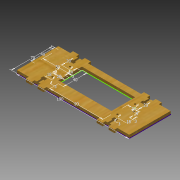
# Autodesk Inventor part: lateral_mdf2
Saved by Autodesk Inventor 2014 (Build 180170000, 170)
## iProperties
Created: 2014-11-10
Part Number: lateral_mdf2
Material: Generic
Document SubType Name: Modeling
Designer: Gabriel
Density: 1 g/cm^3
Appearance: Default
Author: Gabriel
Autodesk Inventor part; units mm, degrees
ref_plane "YZ Plane" through (0, 0, 0) normal (1, 0, 0) x (0, 1, 0)
ref_plane "XZ Plane" through (0, 0, 0) normal (0, 1, 0) x (-1, 0, 0)
ref_plane "XY Plane" through (0, 0, 0) normal (0, 0, 1) x (1, 0, 0)
sketch "Sketch1" plane through (0, 0, 0) normal (0, 0, 1) x (1, 0, 0)
  line L0 (0, 0) -> (190, 0)
  line L1 (190, 0) -> (190, -70)
  line L2 (190, -70) -> (0, -70)
  line L3 (0, -70) -> (0, 0)
  line L4 (0, 0) -> (0, -40)
  line L5 (0, 0) -> (0, -10)
  line L6 (50, -10) -> (50, -50)
  line L7 (50, -50) -> (140, -50)
  line L8 (140, -50) -> (140, -10)
  line L9 (140, -10) -> (50, -10)
  circle A0 centre (40, -20) radius 1.5
  circle A1 centre (150, -20) radius 1.5
  circle A2 centre (150, -50) radius 1.5
  circle A3 centre (40, -50) radius 1.5
  line L10 (50, -10) -> (50, -12)
  line L11 (50, -12) -> (50, -32)
  line L12 (50, -32) -> (30, -32)
  line L13 (140, -32) -> (160, -32)
  circle A4 centre (30, -32) radius 1.5
  circle A5 centre (160, -32) radius 1.5
  dimension "d0" = 190
  dimension "d1" = 70
  dimension "d116" = 40
  dimension "d118" = 50
  dimension "d119" = 40
  dimension "d120" = 90
  dimension "d125" = 3
  dimension "d126" = 3
  dimension "d127" = 3
  dimension "d128" = 3
  dimension "d130" = 20
  dimension "d131" = 20
  dimension "d132" = 20
  dimension "d133" = 3
  dimension "d134" = 3
  dimension "d140" = 20
  dimension "d141" = 20
  dimension "d145" = 18
  dimension "d146" = 18
  constraints: 28 end point, 6 centre point, 5 point on line, 4 parallel, 2 coincident, 2 perpendicular, 1 collinear, 1 horizontal
  measures "d0" distance of L1.end L2.end
  measures "d1" distance of L2.end L0.start
  measures "d116" distance of L0.start L4.end
  measures "d118" distance of L5.end L6.start
  measures "d119" distance of L6.start L6.end
  measures "d120" distance of L6.end L7.end
  measures "d125" diameter of A0
  measures "d126" diameter of A1
  measures "d127" diameter of A2
  measures "d128" diameter of A3
  measures "d130" distance of L10.end L11.end
  measures "d131" distance of L11.end L12.end
  measures "d132" distance of L13.start L13.end
  measures "d133" diameter of A4
  measures "d134" diameter of A5
  measures "d140" distance from line of L0 A0.centre
  measures "d141" distance from line of L0 A1.centre
  measures "d145" distance from line of A2.centre L13
  measures "d146" distance from line of A3.centre L12
extrude "Extrusion3" add sketch "Sketch1" along normal blind 5 contours L0 L1 L2 L3 | L9 L8 L7 L6 | A0 | A1 | A2 | A3 | A4 | A5
sketch "Sketch3" plane through (0, 0, 0) normal (0, 0, -1) x (-1, 0, 0)
  line L0 (0, 0) -> (-35, 0)
  line L1 (-35, 0) -> (-35, -13)
  line L2 (-35, -13) -> (-31.5, -13)
  line L3 (-35, -13) -> (-38.5, -13)
  line L4 (-38.5, -13) -> (-38.5, -8)
  line L5 (-38.5, -8) -> (-36.5, -8)
  line L6 (-36.5, -8) -> (-36.5, 0)
  line L7 (-31.5, -13) -> (-31.5, -8)
  line L8 (-31.5, -8) -> (-33.5, -8)
  line L9 (-33.5, -8) -> (-33.5, 0)
  line L10 (-35, 0) -> (-75, 0) construction
  line L11 (-75, 0) -> (-75, -13)
  line L12 (-75, -13) -> (-71.5, -13)
  line L13 (-75, -13) -> (-78.5, -13)
  line L14 (-78.5, -13) -> (-78.5, -8)
  line L15 (-78.5, -8) -> (-76.5, -8)
  line L16 (-71.5, -13) -> (-71.5, -8)
  line L17 (-71.5, -8) -> (-73.5, -8)
  line L18 (-73.5, -8) -> (-73.5, 0)
  line L19 (-76.5, -8) -> (-76.5, 0)
  line L20 (0, 0) -> (-190, 0) projected
  line L21 (-75, 0) -> (-115, 0)
  line L22 (-115, 0) -> (-115, -13)
  line L23 (-115, -13) -> (-111.5, -13)
  line L24 (-111.5, -13) -> (-111.5, -8)
  line L25 (-111.5, -8) -> (-113.5, -8)
  line L26 (-113.5, -8) -> (-113.5, 0)
  line L27 (-115, -13) -> (-118.5, -13)
  line L28 (-118.5, -13) -> (-118.5, -8)
  line L29 (-118.5, -8) -> (-116.5, -8)
  line L30 (-116.5, -8) -> (-116.5, 0)
  line L31 (-115, 0) -> (-155, 0)
  line L32 (-155, 0) -> (-155, -13)
  line L33 (-155, -13) -> (-151.5, -13)
  line L34 (-151.5, -13) -> (-151.5, -8)
  line L35 (-151.5, -8) -> (-153.5, -8)
  line L36 (-153.5, -8) -> (-153.5, 0)
  line L37 (-155, -13) -> (-158.5, -13)
  line L38 (-158.5, -13) -> (-158.5, -8)
  line L39 (-158.5, -8) -> (-156.5, -8)
  line L40 (-156.5, -8) -> (-156.5, 0)
  line L41 (-76.5, 0) -> (-73.5, 0)
  line L42 (-33.5, -8) -> (-31.5, -8)
  line L43 (-36.5, 0) -> (-33.5, 0)
  line L44 (-155, 0) -> (-155, -70)
  line L45 (-115, 0) -> (-115, -70)
  line L46 (-75, 0) -> (-75, -70)
  line L47 (-35, 0) -> (-35, -70)
  line L48 (-155, -70) -> (-153.5, -70)
  line L49 (-153.5, -70) -> (-153.5, -62)
  line L50 (-153.5, -62) -> (-151.5, -62)
  line L51 (-151.5, -62) -> (-151.5, -57)
  line L52 (-151.5, -57) -> (-155, -57)
  line L53 (-155, -70) -> (-156.5, -70)
  line L54 (-156.5, -70) -> (-156.5, -62)
  line L55 (-156.5, -62) -> (-158.5, -62)
  line L56 (-158.5, -62) -> (-158.5, -57)
  line L57 (-158.5, -57) -> (-155, -57)
  line L58 (-115, -70) -> (-113.5, -70)
  line L59 (-113.5, -70) -> (-113.5, -62)
  line L60 (-113.5, -62) -> (-111.5, -62)
  line L61 (-111.5, -62) -> (-111.5, -57)
  line L62 (-111.5, -57) -> (-115, -57)
  line L63 (-115, -70) -> (-116.5, -70)
  line L64 (-116.5, -70) -> (-116.5, -62)
  line L65 (-116.5, -62) -> (-118.5, -62)
  line L66 (-118.5, -62) -> (-118.5, -57)
  line L67 (-118.5, -57) -> (-115, -57)
  line L68 (-75, -70) -> (-73.5, -70)
  line L69 (-73.5, -70) -> (-73.5, -62)
  line L70 (-73.5, -62) -> (-71.5, -62)
  line L71 (-71.5, -62) -> (-71.5, -57)
  line L72 (-71.5, -57) -> (-75, -57)
  line L73 (-75, -70) -> (-76.5, -70)
  line L74 (-76.5, -70) -> (-76.5, -62)
  line L75 (-76.5, -62) -> (-78.5, -62)
  line L76 (-78.5, -62) -> (-78.5, -57)
  line L77 (-78.5, -57) -> (-75, -57)
  line L78 (-35, -70) -> (-33.5, -70)
  line L79 (-33.5, -70) -> (-33.5, -62)
  line L80 (-33.5, -62) -> (-31.5, -62)
  line L81 (-31.5, -62) -> (-31.5, -57)
  line L82 (-31.5, -57) -> (-38.5, -57)
  line L83 (-38.5, -57) -> (-38.5, -62)
  line L84 (-38.5, -62) -> (-36.5, -62)
  line L85 (-36.5, -62) -> (-36.5, -70)
  line L86 (-36.5, -70) -> (-35, -70)
  dimension "d14" = 35
  dimension "d15" = 13
  dimension "d16" = 3.5
  dimension "d17" = 3.5
  dimension "d18" = 5
  dimension "d19" = 2
  dimension "d20" = 2
  dimension "d21" = 40
  dimension "d22" = 13
  dimension "d23" = 3.5
  dimension "d24" = 3.5
  dimension "d25" = 5
  dimension "d26" = 2
  dimension "d27" = 2
  dimension "d28" = 40
  dimension "d29" = 8
  dimension "d30" = 13
  dimension "d31" = 40
  dimension "d32" = 13
  dimension "d33" = 3.5
  dimension "d34" = 5
  dimension "d35" = 2
  dimension "d36" = 3.5
  dimension "d37" = 5
  dimension "d38" = 2
  dimension "d39" = 40
  dimension "d40" = 13
  dimension "d41" = 3.5
  dimension "d42" = 5
  dimension "d43" = 2
  dimension "d44" = 3.5
  dimension "d45" = 5
  dimension "d46" = 2
  dimension "d63" = 8
  dimension "d66" = 1.5
  dimension "d67" = 5
  dimension "d68" = 1.5
  dimension "d69" = 2
  dimension "d70" = 5
  dimension "d71" = 1.5
  dimension "d72" = 2
  dimension "d73" = 8
  dimension "d74" = 2
  dimension "d75" = 1.5
  constraints: 172 end point, 42 perpendicular, 37 parallel, 12 point on line, 3 collinear, 2 horizontal
  measures "d14" distance of L0.start L0.end
  measures "d15" distance of L0.end L1.end
  measures "d16" distance of L1.end L2.end
  measures "d17" distance of L1.end L3.end
  measures "d18" distance of L3.end L4.end
  measures "d19" distance of L4.end L5.end
  measures "d20" distance of L7.end L8.end
  measures "d21" distance of L10.start L10.end
  measures "d22" distance of L10.end L13.start
  measures "d23" distance of L13.start L16.start
  measures "d24" distance of L13.start L14.start
  measures "d25" distance of L14.start L15.start
  measures "d26" distance of L15.start L15.end
  measures "d27" distance of L17.start L18.start
  measures "d28" distance between parallel lines of L1 L11
  measures "d29" distance of L18.start L18.end
  measures "d30" distance from line of L20 L16.start
  measures "d31" distance of L10.end L21.end
  measures "d32" distance of L21.end L22.end
  measures "d33" distance of L22.end L23.end
  measures "d34" distance of L23.end L24.end
  measures "d35" distance of L24.end L25.end
  measures "d36" distance of L22.end L27.end
  measures "d37" distance of L27.end L28.end
  measures "d38" distance of L28.end L29.end
  measures "d39" distance of L21.end L31.end
  measures "d40" distance of L31.end L32.end
  measures "d41" distance of L32.end L33.end
  measures "d42" distance of L33.end L34.end
  measures "d43" distance of L34.end L35.end
  measures "d44" distance of L32.end L37.end
  measures "d45" distance of L37.end L38.end
  measures "d46" distance of L38.end L39.end
  measures "d63" distance of L48.end L49.end
  measures "d66" distance of L44.end L48.end
  measures "d67" distance of L50.end L51.end
  measures "d68" distance of L44.end L53.end
  measures "d69" distance of L59.end L60.end
  measures "d70" distance of L60.end L61.end
  measures "d71" distance of L45.end L63.end
  measures "d72" distance of L64.end L65.end
  measures "d73" distance of L68.end L69.end
  measures "d74" distance of L69.end L70.end
  measures "d75" distance of L46.end L73.end
extrude "Extrusion4" cut sketch "Sketch3" against normal blind 5 contours L32 L37 L38 L39 L40 L20
extrude "Extrusion5" cut sketch "Sketch3" against normal blind 5 contours L36 L35 L34 L33 L32 L20
extrude "Extrusion9" cut sketch "Sketch3" against normal blind 5 contours L9 L8 L7 L2 L1 L0
extrude "Extrusion10" cut sketch "Sketch3" against normal blind 5 contours L1 L3 L4 L5 L6 L20
extrude "Extrusion11" cut sketch "Sketch3" against normal blind 5 contours L44 L53 L54 L55 L56 L57
extrude "Extrusion12" cut sketch "Sketch3" against normal blind 5 contours L52 L51 L50 L49 L48 L44
extrude "Extrusion17" cut sketch "Sketch3" against normal blind 5 contours L82 L81 L80 L79 L78 L47 | L47 L86 L85 L84 L83 L82
sketch "Sketch4" plane through (153.5, -70, 0) normal (0, -1, 0) x (1, 0, 0)
  line L0 (-153.5, 0) -> (-133.5, 0)
  line L1 (-133.5, 0) -> (-133.5, 5)
  line L2 (-133.5, 5) -> (-123.5, 5)
  line L3 (-123.5, 5) -> (-123.5, 0)
  line L4 (-123.5, 0) -> (-133.5, 0)
  line L5 (-123.5, 5) -> (-113.5, 5)
  line L6 (-113.5, 5) -> (-113.5, 0)
  line L7 (-113.5, 0) -> (-103.5, 0)
  line L8 (-103.5, 0) -> (-103.5, 5)
  line L9 (-103.5, 5) -> (-113.5, 5)
  line L10 (-153.5, 0) -> (36.5, 0)
  line L11 (36.5, 0) -> (16.5, 0)
  line L12 (16.5, 0) -> (16.5, 5)
  line L13 (16.5, 5) -> (6.5, 5)
  line L14 (6.5, 5) -> (6.5, 0)
  line L15 (6.5, 0) -> (-3.5, 0)
  line L16 (-3.5, 0) -> (-3.5, 5)
  line L17 (-3.5, 5) -> (-13.5, 5)
  line L18 (-13.5, 5) -> (-13.5, 0)
  dimension "d90" = 20
  dimension "d91" = 5
  dimension "d92" = 10
  dimension "d93" = 10
  dimension "d94" = 10
  dimension "d95" = 190
  dimension "d96" = 20
  dimension "d97" = 10
  dimension "d98" = 10
  dimension "d99" = 10
  constraints: 38 end point, 8 parallel, 7 perpendicular, 4 point on line, 1 collinear, 1 horizontal
  measures "d90" distance of L0.start L0.end
  measures "d91" distance of L0.end L1.end
  measures "d92" distance of L1.end L2.end
  measures "d93" distance of L2.end L5.end
  measures "d94" distance of L6.end L7.end
  measures "d95" distance of L0.start L10.end
  measures "d96" distance of L10.end L11.end
  measures "d97" distance of L12.end L13.end
  measures "d98" distance of L14.end L15.end
  measures "d99" distance of L16.end L17.end
extrude "Extrusion18" add sketch "Sketch4" along normal blind 5 contours L1 L2 L3 L4 | L6 L9 L8 L7 | L18 L17 L16 L10 | L14 L13 L12 L10
sketch "Sketch5" plane through (190, 0, 5) normal (0, 1, 0) x (1, 0, 0)
  line L0 (-190, 5) -> (-170, 5)
  line L1 (-170, 5) -> (-170, 0)
  line L2 (-170, 0) -> (-160, 0)
  line L3 (-160, 0) -> (-160, 5)
  line L4 (-160, 5) -> (-170, 5)
  line L5 (-160, 5) -> (-150, 5)
  line L6 (-150, 5) -> (-150, 0)
  line L7 (-150, 0) -> (-140, 0)
  line L8 (-140, 0) -> (-140, 5)
  line L9 (-140, 5) -> (-150, 5)
  line L10 (-190, 5) -> (0, 5)
  line L11 (0, 5) -> (-20, 5)
  line L12 (-20, 5) -> (-20, 0)
  line L13 (-20, 0) -> (-30, 0)
  line L14 (-30, 0) -> (-30, 5)
  line L15 (-30, 5) -> (-40, 5)
  line L16 (-40, 5) -> (-40, 0)
  line L17 (-40, 0) -> (-50, 0)
  line L18 (-50, 0) -> (-50, 5)
  dimension "d102" = 20
  dimension "d103" = 5
  dimension "d104" = 10
  dimension "d105" = 10
  dimension "d106" = 10
  dimension "d107" = 190
  dimension "d108" = 20
  dimension "d109" = 5
  dimension "d110" = 10
  dimension "d111" = 10
  dimension "d112" = 5
  dimension "d113" = 10
  constraints: 38 end point, 8 perpendicular, 5 parallel, 4 point on line, 3 collinear, 1 horizontal
  measures "d102" distance of L0.start L0.end
  measures "d103" distance of L0.end L1.end
  measures "d104" distance of L1.end L2.end
  measures "d105" distance of L3.end L5.end
  measures "d106" distance of L6.end L7.end
  measures "d107" distance of L0.start L10.end
  measures "d108" distance of L10.end L11.end
  measures "d109" distance of L11.end L12.end
  measures "d110" distance of L12.end L13.end
  measures "d111" distance of L14.end L15.end
  measures "d112" distance of L15.end L16.end
  measures "d113" distance of L16.end L17.end
extrude "Extrusion19" add sketch "Sketch5" along normal blind 5
extrude "Extrusion20" cut sketch "Sketch1" along normal blind 10 contours L9 L8 L7 L6
extrude "Extrusion22" cut sketch "Sketch1" along normal blind 10 contours A0 | A1 | A2 | A3 | A4 | A5
body "Solid2"
